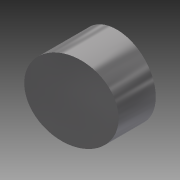
# Autodesk Inventor part: tungsten
Saved by Autodesk Inventor 2015 (Build 190159000, 159)
## iProperties
Created: 2014-09-24
Part Number: tungsten
Material: Steel, Mild
Document SubType Name: Modeling
Designer: Adam
Density: 7.85 g/cm^3
Appearance: Semi-Polished
Author: Adam
Autodesk Inventor part; units mm, degrees
ref_plane "YZ Plane" through (0, 0, 0) normal (1, 0, 0) x (0, 1, 0)
sketch "Sketch1" plane through (0, 0, 0) normal (0, 0, 1) x (1, 0, 0)
  circle A0 centre (0, 0) radius 6 projected
  point P0 (0, 0)
ref_plane "Work Plane1" through (-7.3084, -8, 8.5534) normal (0.2079117, 0, 0.9781476) x (0.9781476, 0, -0.2079117)
ref_plane "Work Plane2" through (-7.3084, -8, 7.5534) normal (0.2079117, 0, 0.9781476) x (0.9781476, 0, -0.2079117)
extrude "Extrusion1" add sketch "Sketch1" along normal up to surface surface through (-7.3084, -8, 7.5534) normal (0.2079117, 0, 0.9781476)
ref_plane "Work Plane3" through (0, 0, 6.8) normal (0, 0, 1) x (1, 0, 0)
sketch "Sketch2" plane through (0, 0, 6.8) normal (0, 0, 1) x (1, 0, 0)
  circle A0 centre (0, 0) radius 10
  dimension "d2" = 20
  constraints: 1 centre point, 1 coincident
  measures "d2" diameter of A0
extrude "Extrusion2" cut sketch "Sketch2" along normal through all
fillet_without_effect "Fillet1"
body "Solid1"
